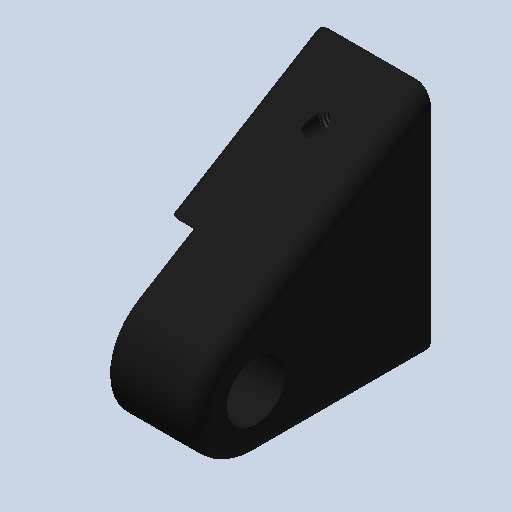
# Autodesk Inventor part: MOUNT,SPRING,ELEVATOR
Saved by Autodesk Inventor 2025.2 (Build 292293000, 293)
## iProperties
Category: _
Manager: _
ILogicPurgeVersion: 0.0.0.0
OnSaveVersion: 3.4.3.0
OnSaveAssembly: COREAutomationManager
Created: 2025-02-07
Part Number: MOUNT,SPRING,ELEVATOR
Checked By: 00
Engr Approved By: _
User Status: Work In Process
Material: 3D Print Material - chopped carbon Nylon12 (preferred)
Description: STANDARD (mm)
Document SubType Name: Modeling
Mfg Approved By: John.Thibert
Designer: John.Thibert
Manufacturer: Standard
Standards Organization: Custom
Mass: 37.9764 g
Surface Area: 86.2808 cm^2
Volume: 36.1048 cm^3
Density: 1.05184 g/cm^3
Appearance: Black
CN_MASS: 0.04
CN_SERVICEABLE: _
FIRST_DESCRIPTION: _
SECOND_DESCRIPTION: _
THIRD_DESCRIPTION: _
ModelCat: Uncategorized
MaterialName: 3D Print Material - chopped carbon Nylon12 (preferred)
Subject: _
Author: John.Thibert
Keywords: -
Revision Number: A
Autodesk Inventor part; units mm, degrees
ref_plane "YZ Plane" through (0, 0, 0) normal (1, 0, 0) x (0, 1, 0)
ref_plane "XZ Plane" through (0, 0, 0) normal (0, 1, 0) x (-1, 0, 0)
ref_plane "XY Plane" through (0, 0, 0) normal (0, 0, 1) x (1, 0, 0)
sketch "Sketch2" plane through (0, 0, 0) normal (1, 0, 0) x (0, 1, 0)
  arc A0 (10.8439, 6.6106) -> (-12.7, 0) centre (0, 0) ccw
  line L0 (10.8439, 6.6106) -> (38.1, -38.1)
  line L1 (38.1, -38.1) -> (-12.7, -38.1)
  line L2 (-12.7, -38.1) -> (-12.7, 0)
  line L3 (-25.8661, 0) -> (48.761, 0) construction
  dimension "d0" = 12.7
  dimension "d1" = 50.8
  dimension "d2" = 38.1
  constraints: 6 end point, 2 point on circle, 2 tangent, 1 centre point, 1 coincident, 1 horizontal, 1 vertical
  measures "d0" radius of A0
  measures "d1" distance of L0.end L1.end
  measures "d2" distance between parallel lines of L3 L1
extrude "Extrusion1" add sketch "Sketch2" along normal mid plane 25.4
sketch "Sketch4" plane through (12.7, 0, 0) normal (1, 0, 0) x (0, 0, -1)
  point P0 (0, 0)
  point P1 (0, 0)
  constraints: 1 coincident
hole "Hole1" at (12.7, 0, 0) direction (-1, 0, 0) diameter 12.7 end through all
sketch "Sketch3" plane through (-12.7, 0, 0) normal (-1, 0, 0) x (0, 0, 1)
  arc A0 (-5.5133, 18.2348) -> (-19.05, 0) centre (0, 0) ccw
  circle A1 centre (0, 0) radius 6.35 construction
  arc A2 (0, -12.7) -> (6.6106, 10.8439) centre (0, 0) ccw projected
  line L0 (6.6106, 10.8439) -> (-38.1, 38.1) projected
  line L1 (-38.1, 38.1) -> (-38.1, -12.7) construction
  line L2 (-38.1, -12.7) -> (0, -12.7) projected
  line L3 (-19.05, 0) -> (-19.05, -12.7)
  dimension "d5" = 38.1
  constraints: 2 end point, 2 point on circle, 1 centre point, 1 coincident, 1 midpoint, 1 perpendicular, 1 point on line
  measures "d5" diameter of A0
extrude "Extrusion2" cut sketch "Sketch3" against normal blind 6.35
sketch "Sketch5" plane through (12.7, 38.1, -38.1) normal (0, 0, -1) x (-1, 0, 0)
  line L0 (12.7, -60.96) -> (12.7, 10.16) construction
  point P0 (12.7, -38.1)
  point P1 (12.7, -46.0375)
  dimension "d15" = 7.9375
  constraints: 1 point on line
  measures "d15" distance of point (12.7, -38.1) point (12.7, -46.037)
hole "Hole2" at (0, -7.9375, -38.1) direction (0, 0, 1) diameter 3.9624 depth 13.6144 tip angle 118 thread size "10-32 UNF" class "2B" standard "ANSI Unified Screw Threads"
pattern_linear "Rectangular Pattern1" count 4 spacing 12.7 along (0, 1, 0) of "Hole2"
fillet "Fillet1" radius 3.175 5 edges at (12.7, -3.4331, 12.2272) (12.7, -12.7, -19.05) (12.7, 24.472, -15.7447) (-12.7, 28.1674, -21.8066) (-12.7, -12.7, -28.575)
body "Solid1"
